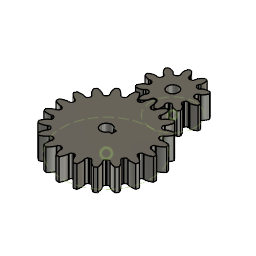
Spur gear (Autodesk Fusion 360 design; units mm, degrees)
part number: 2026-06-27-18-00-24-643
description: Spur Gear; Module: 2.0; Num Teeth: 20; Pressure Angle: 20.0; Backlash: 0.00 mm
part number: 2026-06-27-18-05-55-851
description: Spur Gear; Module: 2.0; Num Teeth: 10; Pressure Angle: 20.0; Backlash: 0.00 mm
part number: 2026-06-27-18-27-18-018
Autodesk Fusion 360 part; units mm, degrees
sketch "Base Circle" plane through (0, 0, 0) normal (0, 0, 1) x (1, 0, 0) in component "Spur Gear 20 teeth"
  circle A0 centre (0, 0) radius 17.686
  line L0 (3.5, 1) -> (2.2913, 1)
  line L1 (2.2913, -1) -> (3.5, -1)
  line L2 (3.5, -1) -> (3.5, 1)
  arc A1 (2.2913, 1) -> (2.2913, -1) centre (0, 0) ccw
  constraint horizontal L0
  constraint parallel L0 L1
extrude "Extrude1" add sketch "Base Circle" along normal blind 10 makes body 1 in component "Spur Gear 20 teeth"
sketch "Gear Tooth" plane through (0, 0, 0) normal (0, 0, 1) x (1, 0, 0) in component "Spur Gear 20 teeth"
  spline S0 degree 5 poles (18.7119, -1.7536) (18.7212, -1.7545) (18.74, -1.756) (18.7682, -1.7575) (18.8059, -1.7581) (18.853, -1.7569) (18.9002, -1.7543) (18.9474, -1.7508) (18.9947, -1.7468) (19.042, -1.7426) (19.0893, -1.738) (19.1367, -1.7329) (19.184, -1.7273) (19.2314, -1.721) (19.2787, -1.714) (19.3261, -1.7063) (19.3735, -1.6982) (19.4208, -1.6895) (19.4682, -1.6805) (19.5156, -1.6711) (19.5629, -1.6613) (19.6103, -1.6511) (19.6576, -1.6405) (19.7049, -1.6295) (19.7522, -1.6181) (19.7995, -1.6062) (19.8468, -1.594) (19.8941, -1.5814) (19.9413, -1.5684) (19.9886, -1.5551) (20.0358, -1.5415) (20.083, -1.5275) (20.1302, -1.5131) (20.1773, -1.4984) (20.2244, -1.4834) (20.2716, -1.4681) (20.3186, -1.4524) (20.3657, -1.4364) (20.4127, -1.42) (20.4597, -1.4034) (20.5067, -1.3865) (20.5536, -1.3692) (20.6005, -1.3517) (20.6474, -1.3338) (20.6942, -1.3156) (20.741, -1.2972) (20.7878, -1.2784) (20.8345, -1.2594) (20.8812, -1.24) (20.9279, -1.2204) (20.9745, -1.2005) (21.0211, -1.1803) (21.0676, -1.1599) (21.1141, -1.1391) (21.1606, -1.1181) (21.207, -1.0968) (21.2534, -1.0753) (21.2997, -1.0534) (21.346, -1.0313) (21.3923, -1.009) (21.4385, -0.9864) (21.4846, -0.9635) (21.5307, -0.9403) (21.5768, -0.9169) (21.6228, -0.8932) (21.6688, -0.8693) (21.7147, -0.8451) (21.7605, -0.8207) (21.8063, -0.796) (21.8521, -0.7711) (21.8978, -0.7459) (21.9343, -0.7256) (21.9617, -0.7102) (21.9799, -0.6999) (21.989, -0.6948) knots 0 0 0 0 0 0 0.01428571 0.02857143 0.04285714 0.05714286 0.07142857 0.08571429 0.1 0.11428571 0.12857143 0.14285714 0.15714286 0.17142857 0.18571429 0.2 0.21428571 0.22857143 0.24285714 0.25714286 0.27142857 0.28571429 0.3 0.31428571 0.32857143 0.34285714 0.35714286 0.37142857 0.38571429 0.4 0.41428571 0.42857143 0.44285714 0.45714286 0.47142857 0.48571429 0.5 0.51428571 0.52857143 0.54285714 0.55714286 0.57142857 0.58571429 0.6 0.61428571 0.62857143 0.64285714 0.65714286 0.67142857 0.68571429 0.7 0.71428571 0.72857143 0.74285714 0.75714286 0.77142857 0.78571429 0.8 0.81428571 0.82857143 0.84285714 0.85714286 0.87142857 0.88571429 0.9 0.91428571 0.92857143 0.94285714 0.95714286 0.97142857 0.98571429 1 1 1 1 1 1
  spline S1 degree 5 poles (18.7119, 1.7536) (18.7212, 1.7545) (18.74, 1.756) (18.7682, 1.7575) (18.8059, 1.7581) (18.853, 1.7569) (18.9002, 1.7543) (18.9474, 1.7508) (18.9947, 1.7468) (19.042, 1.7426) (19.0893, 1.738) (19.1367, 1.7329) (19.184, 1.7273) (19.2314, 1.721) (19.2787, 1.714) (19.3261, 1.7063) (19.3735, 1.6982) (19.4208, 1.6895) (19.4682, 1.6805) (19.5156, 1.6711) (19.5629, 1.6613) (19.6103, 1.6511) (19.6576, 1.6405) (19.7049, 1.6295) (19.7522, 1.6181) (19.7995, 1.6062) (19.8468, 1.594) (19.8941, 1.5814) (19.9413, 1.5684) (19.9886, 1.5551) (20.0358, 1.5415) (20.083, 1.5275) (20.1302, 1.5131) (20.1773, 1.4984) (20.2244, 1.4834) (20.2716, 1.4681) (20.3186, 1.4524) (20.3657, 1.4364) (20.4127, 1.42) (20.4597, 1.4034) (20.5067, 1.3865) (20.5536, 1.3692) (20.6005, 1.3517) (20.6474, 1.3338) (20.6942, 1.3156) (20.741, 1.2972) (20.7878, 1.2784) (20.8345, 1.2594) (20.8812, 1.24) (20.9279, 1.2204) (20.9745, 1.2005) (21.0211, 1.1803) (21.0676, 1.1599) (21.1141, 1.1391) (21.1606, 1.1181) (21.207, 1.0968) (21.2534, 1.0753) (21.2997, 1.0534) (21.346, 1.0313) (21.3923, 1.009) (21.4385, 0.9864) (21.4846, 0.9635) (21.5307, 0.9403) (21.5768, 0.9169) (21.6228, 0.8932) (21.6688, 0.8693) (21.7147, 0.8451) (21.7605, 0.8207) (21.8063, 0.796) (21.8521, 0.7711) (21.8978, 0.7459) (21.9343, 0.7256) (21.9617, 0.7102) (21.9799, 0.6999) (21.989, 0.6948) knots 0 0 0 0 0 0 0.01428571 0.02857143 0.04285714 0.05714286 0.07142857 0.08571429 0.1 0.11428571 0.12857143 0.14285714 0.15714286 0.17142857 0.18571429 0.2 0.21428571 0.22857143 0.24285714 0.25714286 0.27142857 0.28571429 0.3 0.31428571 0.32857143 0.34285714 0.35714286 0.37142857 0.38571429 0.4 0.41428571 0.42857143 0.44285714 0.45714286 0.47142857 0.48571429 0.5 0.51428571 0.52857143 0.54285714 0.55714286 0.57142857 0.58571429 0.6 0.61428571 0.62857143 0.64285714 0.65714286 0.67142857 0.68571429 0.7 0.71428571 0.72857143 0.74285714 0.75714286 0.77142857 0.78571429 0.8 0.81428571 0.82857143 0.84285714 0.85714286 0.87142857 0.88571429 0.9 0.91428571 0.92857143 0.94285714 0.95714286 0.97142857 0.98571429 1 1 1 1 1 1
  arc A0 (21.989, -0.6948) -> (21.989, 0.6948) centre (0, 0) ccw
  line L0 (17.5989, -1.6493) -> (18.7119, -1.7536)
  line L1 (17.5989, 1.6493) -> (18.7119, 1.7536)
  line L2 (17.5989, -1.6493) -> (17.5989, 1.6493)
  point P0 (18.9421, -1.7511)
  point P1 (19.1741, -1.7283)
  point P2 (19.4073, -1.6919)
  point P3 (19.6412, -1.6441)
  point P4 (19.8757, -1.5862)
  point P5 (20.1106, -1.519)
  point P6 (20.3458, -1.4431)
  point P7 (20.5811, -1.3589)
  point P8 (20.8164, -1.2667)
  point P9 (21.0516, -1.1669)
  point P10 (21.2866, -1.0596)
  point P11 (21.5212, -0.945)
  point P12 (21.7554, -0.8234)
  point P13 (18.9421, 1.7511)
  point P14 (19.1741, 1.7283)
  point P15 (19.4073, 1.6919)
  point P16 (19.6412, 1.6441)
  point P17 (19.8757, 1.5862)
  point P18 (20.1106, 1.519)
  point P19 (20.3458, 1.4431)
  point P20 (20.5811, 1.3589)
  point P21 (20.8164, 1.2667)
  point P22 (21.0516, 1.1669)
  point P23 (21.2866, 1.0596)
  point P24 (21.5212, 0.945)
  point P25 (21.7554, 0.8234)
extrude "Extrude2" add sketch "Gear Tooth" along normal blind 10 bodies 1 in component "Spur Gear 20 teeth"
fillet "Fillet1" radius 1 2 edges at (17.6088, -1.6503, 5) (17.6088, 1.6503, 5) on bodies 1 in component "Spur Gear 20 teeth"
pattern_circular "C-Pattern1" count 20 over 360 about axis through (0, 0, 0) along (0, 0, 1) of "Extrude2", "Fillet1" in component "Spur Gear 20 teeth"
sketch "Base Circle (2)" plane through (0, 0, 0) normal (0, 0, 1) x (1, 0, 0) in component "Spur Gear 10 teeth"
  circle A0 centre (0, 0) radius 7.686
  circle A1 centre (0, 0) radius 2.5
extrude "Extrude1'" add sketch "Base Circle (2)" along normal blind 10 separate body makes body 2 in component "Spur Gear 10 teeth"
sketch "Gear Tooth (2)" plane through (0, 0, 0) normal (0, 0, 1) x (1, 0, 0) in component "Spur Gear 10 teeth"
  spline S0 degree 5 poles (9.2583, -1.6082) (9.2659, -1.6095) (9.2813, -1.6119) (9.3043, -1.6147) (9.3352, -1.6169) (9.374, -1.6176) (9.413, -1.6169) (9.4522, -1.6152) (9.4913, -1.6131) (9.5306, -1.6106) (9.5699, -1.6078) (9.6092, -1.6044) (9.6485, -1.6005) (9.688, -1.5957) (9.7275, -1.5903) (9.767, -1.5842) (9.8065, -1.5774) (9.8461, -1.5702) (9.8857, -1.5626) (9.9253, -1.5546) (9.9649, -1.5461) (10.0045, -1.5372) (10.0441, -1.5278) (10.0838, -1.5179) (10.1234, -1.5076) (10.163, -1.4969) (10.2027, -1.4857) (10.2423, -1.4741) (10.2819, -1.4621) (10.3215, -1.4497) (10.3611, -1.4369) (10.4006, -1.4237) (10.4402, -1.4102) (10.4797, -1.3962) (10.5192, -1.3819) (10.5587, -1.3672) (10.5982, -1.3521) (10.6376, -1.3367) (10.677, -1.3209) (10.7163, -1.3047) (10.7557, -1.2882) (10.795, -1.2713) (10.8342, -1.2541) (10.8734, -1.2366) (10.9126, -1.2187) (10.9517, -1.2004) (10.9908, -1.1818) (11.0298, -1.1629) (11.0688, -1.1437) (11.1078, -1.1241) (11.1466, -1.1042) (11.1855, -1.084) (11.2242, -1.0634) (11.2629, -1.0425) (11.3016, -1.0213) (11.3402, -0.9998) (11.3787, -0.978) (11.4172, -0.9559) (11.4556, -0.9334) (11.4939, -0.9107) (11.5322, -0.8876) (11.5704, -0.8642) (11.6085, -0.8406) (11.6466, -0.8166) (11.6846, -0.7923) (11.7225, -0.7677) (11.7603, -0.7429) (11.7981, -0.7177) (11.8358, -0.6923) (11.8733, -0.6665) (11.9109, -0.6405) (11.9408, -0.6194) (11.9632, -0.6035) (11.9781, -0.5928) (11.9856, -0.5875) knots 0 0 0 0 0 0 0.01428571 0.02857143 0.04285714 0.05714286 0.07142857 0.08571429 0.1 0.11428571 0.12857143 0.14285714 0.15714286 0.17142857 0.18571429 0.2 0.21428571 0.22857143 0.24285714 0.25714286 0.27142857 0.28571429 0.3 0.31428571 0.32857143 0.34285714 0.35714286 0.37142857 0.38571429 0.4 0.41428571 0.42857143 0.44285714 0.45714286 0.47142857 0.48571429 0.5 0.51428571 0.52857143 0.54285714 0.55714286 0.57142857 0.58571429 0.6 0.61428571 0.62857143 0.64285714 0.65714286 0.67142857 0.68571429 0.7 0.71428571 0.72857143 0.74285714 0.75714286 0.77142857 0.78571429 0.8 0.81428571 0.82857143 0.84285714 0.85714286 0.87142857 0.88571429 0.9 0.91428571 0.92857143 0.94285714 0.95714286 0.97142857 0.98571429 1 1 1 1 1 1
  spline S1 degree 5 poles (9.2583, 1.6082) (9.2659, 1.6095) (9.2813, 1.6119) (9.3043, 1.6147) (9.3352, 1.6169) (9.374, 1.6176) (9.413, 1.6169) (9.4522, 1.6152) (9.4913, 1.6131) (9.5306, 1.6106) (9.5699, 1.6078) (9.6092, 1.6044) (9.6485, 1.6005) (9.688, 1.5957) (9.7275, 1.5903) (9.767, 1.5842) (9.8065, 1.5774) (9.8461, 1.5702) (9.8857, 1.5626) (9.9253, 1.5546) (9.9649, 1.5461) (10.0045, 1.5372) (10.0441, 1.5278) (10.0838, 1.5179) (10.1234, 1.5076) (10.163, 1.4969) (10.2027, 1.4857) (10.2423, 1.4741) (10.2819, 1.4621) (10.3215, 1.4497) (10.3611, 1.4369) (10.4006, 1.4237) (10.4402, 1.4102) (10.4797, 1.3962) (10.5192, 1.3819) (10.5587, 1.3672) (10.5982, 1.3521) (10.6376, 1.3367) (10.677, 1.3209) (10.7163, 1.3047) (10.7557, 1.2882) (10.795, 1.2713) (10.8342, 1.2541) (10.8734, 1.2366) (10.9126, 1.2187) (10.9517, 1.2004) (10.9908, 1.1818) (11.0298, 1.1629) (11.0688, 1.1437) (11.1078, 1.1241) (11.1466, 1.1042) (11.1855, 1.084) (11.2242, 1.0634) (11.2629, 1.0425) (11.3016, 1.0213) (11.3402, 0.9998) (11.3787, 0.978) (11.4172, 0.9559) (11.4556, 0.9334) (11.4939, 0.9107) (11.5322, 0.8876) (11.5704, 0.8642) (11.6085, 0.8406) (11.6466, 0.8166) (11.6846, 0.7923) (11.7225, 0.7677) (11.7603, 0.7429) (11.7981, 0.7177) (11.8358, 0.6923) (11.8733, 0.6665) (11.9109, 0.6405) (11.9408, 0.6194) (11.9632, 0.6035) (11.9781, 0.5928) (11.9856, 0.5875) knots 0 0 0 0 0 0 0.01428571 0.02857143 0.04285714 0.05714286 0.07142857 0.08571429 0.1 0.11428571 0.12857143 0.14285714 0.15714286 0.17142857 0.18571429 0.2 0.21428571 0.22857143 0.24285714 0.25714286 0.27142857 0.28571429 0.3 0.31428571 0.32857143 0.34285714 0.35714286 0.37142857 0.38571429 0.4 0.41428571 0.42857143 0.44285714 0.45714286 0.47142857 0.48571429 0.5 0.51428571 0.52857143 0.54285714 0.55714286 0.57142857 0.58571429 0.6 0.61428571 0.62857143 0.64285714 0.65714286 0.67142857 0.68571429 0.7 0.71428571 0.72857143 0.74285714 0.75714286 0.77142857 0.78571429 0.8 0.81428571 0.82857143 0.84285714 0.85714286 0.87142857 0.88571429 0.9 0.91428571 0.92857143 0.94285714 0.95714286 0.97142857 0.98571429 1 1 1 1 1 1
  arc A0 (11.9856, -0.5875) -> (11.9856, 0.5875) centre (0, 0) ccw
  line L0 (7.5628, -1.3137) -> (9.2583, -1.6082)
  line L1 (7.5628, 1.3137) -> (9.2583, 1.6082)
  line L2 (7.5628, -1.3137) -> (7.5628, 1.3137)
  point P0 (9.4457, -1.6154)
  point P1 (9.6366, -1.6016)
  point P2 (9.8296, -1.5732)
  point P3 (10.0242, -1.5325)
  point P4 (10.2199, -1.4806)
  point P5 (10.4164, -1.4183)
  point P6 (10.6134, -1.3461)
  point P7 (10.8107, -1.2644)
  point P8 (11.008, -1.1735)
  point P9 (11.205, -1.0736)
  point P10 (11.4014, -0.9649)
  point P11 (11.5972, -0.8476)
  point P12 (11.792, -0.7217)
  point P13 (9.4457, 1.6154)
  point P14 (9.6366, 1.6016)
  point P15 (9.8296, 1.5732)
  point P16 (10.0242, 1.5325)
  point P17 (10.2199, 1.4806)
  point P18 (10.4164, 1.4183)
  point P19 (10.6134, 1.3461)
  point P20 (10.8107, 1.2644)
  point P21 (11.008, 1.1735)
  point P22 (11.205, 1.0736)
  point P23 (11.4014, 0.9649)
  point P24 (11.5972, 0.8476)
  point P25 (11.792, 0.7217)
extrude "Extrude2'" add sketch "Gear Tooth (2)" along normal blind 10 bodies 2 in component "Spur Gear 10 teeth"
fillet "Fillet1'" radius 1 2 edges at (7.5726, -1.3154, 5) (7.5726, 1.3154, 5) on bodies 2 in component "Spur Gear 10 teeth"
pattern_circular "C-Pattern1'" count 10 over 360 about axis through (0, 0, 0) along (0, 0, 1) of "Extrude2'", "Fillet1'" in component "Spur Gear 10 teeth"
sketch "Diametrial Pitch Circle" plane through (0, 0, 0) normal (0, 0, 1) x (1, 0, 0) in component "Spur Gear 10 teeth"
  circle A0 centre (0, 0) radius 10 construction
move_face "MoveFace1" by (0, 30, 0) 1 faces at (1.8662, 5.5821, 10) on bodies 2 in component "Spur Gear 10 teeth"
move_face "MoveFace2" by (0, 39, 0) 1 faces at (1.8662, 5.5821, 10) on bodies 2 in component "Spur Gear 10 teeth"
sketch "Diametrial Pitch Circle (2)" plane through (0, 0, 0) normal (0, 0, 1) x (1, 0, 0) in component "Spur Gear 20 teeth"
  circle A0 centre (0, 0) radius 20 construction
component "Spur Gear 20 teeth" placed x (1, 0, 0) y (0, 1, 0) z (0, 0, 1) at (0, 0, 0)
component "Spur Gear 10 teeth" placed x (1, 0, 0) y (0, 1, 0) z (0, 0, 1) at (0, 0, 0)
